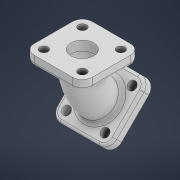
# Autodesk Inventor part: Pieza de practica 6
Saved by Autodesk Inventor 2022 (Build 260153000, 153)
## iProperties
Created: 2022-07-05
Part Number: Pieza de practica 6
Material: Genérico
Document SubType Name: Modeling
Designer: aleon
Density: 1 g/cm^3
Appearance: Valor por defecto
Author: aleon
Autodesk Inventor part; units mm, degrees
ref_plane "YZ Plane" through (0, 0, 0) normal (1, 0, 0) x (0, 1, 0)
ref_plane "XZ Plane" through (0, 0, 0) normal (0, 1, 0) x (-1, 0, 0)
sketch "Boceto1" plane through (0, 0, 0) normal (0, 1, 0) x (-1, 0, 0)
  circle A0 centre (0, 0) radius 44
  circle A1 centre (0, 0) radius 68.5
  line L0 (-74.5, -112.5) -> (74.5, -112.5)
  line L1 (112.5, -74.5) -> (112.5, 74.5)
  line L2 (74.5, 112.5) -> (-74.5, 112.5)
  line L3 (-112.5, 74.5) -> (-112.5, -74.5)
  line L4 (-112.5, -112.5) -> (112.5, 112.5) construction
  line L5 (112.5, -112.5) -> (-112.5, 112.5) construction
  arc A2 (112.5, 74.5) -> (74.5, 112.5) centre (74.5, 74.5) ccw
  arc A3 (74.5, -112.5) -> (112.5, -74.5) centre (74.5, -74.5) ccw
  arc A4 (-112.5, -74.5) -> (-74.5, -112.5) centre (-74.5, -74.5) ccw
  arc A5 (-74.5, 112.5) -> (-112.5, 74.5) centre (-74.5, 74.5) ccw
  circle A6 centre (-74.5, 74.5) radius 16
  circle A7 centre (-74.5, -74.5) radius 16
  circle A8 centre (74.5, -74.5) radius 16
  circle A9 centre (74.5, 74.5) radius 16
  dimension "d0" = 88
  dimension "d1" = 137
  dimension "d6" = 225
  dimension "d7" = 225
  dimension "d8" = 38
  dimension "d11" = 32
  dimension "d12" = 32
  dimension "d13" = 32
  dimension "d14" = 32
  constraints: 12 end point, 10 centre point, 8 point on circle, 8 point on line, 8 tangent, 6 coincident, 3 equal radius, 2 midpoint, 2 parallel, 1 horizontal, 1 perpendicular
  measures "d0" diameter of A0
  measures "d1" diameter of A1
  measures "d6" distance of L5.end L4.end
  measures "d7" distance of L4.end L5.start
  measures "d8" radius of A2
  measures "d11" diameter of A6
  measures "d12" diameter of A7
  measures "d13" diameter of A8
  measures "d14" diameter of A9
sketch "Boceto2" plane through (0, 0, 0) normal (1, 0, 0) x (0, 1, 0)
  line L0 (0, 0) -> (0, -225) construction
  line L1 (0, -225) -> (-379.7593, 154.7593) construction
  arc A0 (0, 0) -> (-159.099, -65.901) centre (0, -225) ccw
  dimension "d2" = 45
  dimension "d3" = 225
  constraints: 5 end point, 2 point on circle, 1 centre point, 1 point on line, 1 vertical
  measures "d2" angle of L1 L0
  measures "d3" radius of A0
sweep "Barrido1" add profiles "Boceto1" path "Boceto2" contours A1
ref_plane "Plano de trabajo1" through (0, 0, -225) normal (0, -0.9238795, -0.3826834) x (1, 0, 0)
extrude "Extrusión2" add sketch "Boceto1" along normal blind 37 contours A1 | A4 L3 A5 L2 A2 L1 A3 L0
fillet "Empalme1" radius 10 8 edges at (101.3701, 0, -101.3701) (0, 0, -112.5) (-101.3701, 0, -101.3701) (-112.5, 0, 0) (-101.3701, 0, 101.3701) (0, 0, 112.5) (101.3701, 0, 101.3701) (112.5, 0, 0)
fillet "Empalme2" radius 15 1 edges at (68.5, 0, 0)
mirror "Simetría1" about plane through (0, 0, -225) normal (0, -0.9238795, -0.3826834) of "Extrusión2", "Empalme1", "Empalme2"
sketch "Boceto3" plane through (74.5, -105.7125, -171.6134) normal (0, -0.7071068, -0.7071068) x (-1, 0, 0)
  circle A0 centre (74.5, -112.5) radius 44 projected
  circle A1 centre (74.5, -112.5) radius 65
  point P0 (74.5, -46.599)
  dimension "d19" = 130
  constraints: 1 centre point, 1 coincident
  measures "d19" diameter of A1
extrude "Extrusión3" add sketch "Boceto3" along normal blind 10
